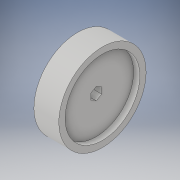
# Autodesk Inventor part: WheelV1
Saved by Autodesk Inventor 2019 (Build 230136000, 136)
## iProperties
Created: 2021-09-16
Part Number: WheelV1
Material: Generic
Document SubType Name: Modeling
Designer: timmy
Density: 1 g/cm^3
Appearance: Default
Author: timmy
Autodesk Inventor part; units mm, degrees
ref_plane "YZ Plane" through (0, 0, 0) normal (1, 0, 0) x (0, 1, 0)
ref_plane "XZ Plane" through (0, 0, 0) normal (0, 1, 0) x (-1, 0, 0)
ref_plane "XY Plane" through (0, 0, 0) normal (0, 0, 1) x (1, 0, 0)
sketch "Sketch1" plane through (0, 0, 0) normal (1, 0, 0) x (0, 1, 0)
  circle A0 centre (0, 0) radius 88.9
  dimension "d0" = 177.8
  constraints: 1 centre point, 1 coincident
  measures "d0" diameter of A0
extrude "Extrusion1" add sketch "Sketch1" along normal blind 50.8
sketch "Sketch2" plane through (50.8, 0, 0) normal (1, 0, 0) x (0, 0, -1)
  circle A0 centre (0, 0) radius 88.9 projected
  circle A1 centre (0, 0) radius 76.2
  dimension "d3" = 12.7
  constraints: 1 centre point
  measures "d3" radial gap between concentric circles of A0 A1
extrude "Extrusion2" cut sketch "Sketch2" against normal blind 12.7 contours A1
sketch "Sketch4" plane through (0, 0, 0) normal (-1, 0, 0) x (0, 0, 1)
  circle A0 centre (0, 0) radius 76.2 projected
extrude "Extrusion3" cut sketch "Sketch4" against normal blind 12.7
sketch "Sketch5" plane through (38.1, 0, 0) normal (1, 0, 0) x (0, 0, -1)
  line L0 (0, 0) -> (0, 12.7)
  line L1 (0, 12.7) -> (10.9985, 6.35)
  line L2 (10.9985, 6.35) -> (10.9985, -6.35)
  line L3 (10.9985, -6.35) -> (0, -12.7)
  line L4 (0, -12.7) -> (-10.9985, -6.35)
  line L5 (-10.9985, -6.35) -> (-10.9985, 6.35)
  line L6 (-10.9985, 6.35) -> (0, 12.7)
  dimension "d8" = 12.7
  constraints: 14 end point, 1 coincident, 1 vertical, 13 other
  measures "d8" distance of L0.start L0.end
extrude "Extrusion4" cut sketch "Sketch5" against normal blind 127
body "Solid1"
